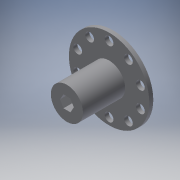
# Autodesk Inventor part: clutch plate
Saved by Autodesk Inventor 2017 (Build 210142000, 142)
## iProperties
Created: 2017-11-23
Part Number: clutch plate
Material: Generic
Document SubType Name: Modeling
Designer: prakh
Density: 1 g/cm^3
Appearance: Default
Author: prakh
Autodesk Inventor part; units mm, degrees
ref_plane "YZ Plane" through (0, 0, 0) normal (1, 0, 0) x (0, 1, 0)
ref_plane "XZ Plane" through (0, 0, 0) normal (0, 1, 0) x (-1, 0, 0)
ref_plane "XY Plane" through (0, 0, 0) normal (0, 0, 1) x (1, 0, 0)
sketch "Sketch1" plane through (0, 0, 0) normal (0, 0, 1) x (1, 0, 0)
  circle A0 centre (0, 0) radius 31.75
  circle A1 centre (0, 26.0608) radius 3.429
  line L0 (2.7496, 4.7625) -> (5.4993, 0)
  line L1 (5.4993, 0) -> (2.7496, -4.7625)
  line L2 (2.7496, -4.7625) -> (-2.7496, -4.7625)
  line L3 (-2.7496, -4.7625) -> (-5.4993, 0)
  line L4 (-5.4993, 0) -> (-2.7496, 4.7625)
  line L5 (-2.7496, 4.7625) -> (2.7496, 4.7625)
  circle A2 centre (-15.3182, 21.0836) radius 3.429
  circle A3 centre (-24.7853, 8.0532) radius 3.429
  circle A4 centre (-24.7853, -8.0532) radius 3.429
  circle A5 centre (-15.3182, -21.0836) radius 3.429
  circle A6 centre (0, -26.0608) radius 3.429
  circle A7 centre (15.3182, -21.0836) radius 3.429
  circle A8 centre (24.7853, -8.0532) radius 3.429
  circle A9 centre (24.7853, 8.0532) radius 3.429
  circle A10 centre (15.3182, 21.0836) radius 3.429
  dimension "d0" = 6.858
  dimension "d1" = 9.525
  dimension "d4" = 360
  dimension "d8" = 63.5
  constraints: 12 end point, 11 centre point, 2 coincident, 34 other
  measures "d0" diameter of A1
  measures "d1" distance between parallel lines of L5 L2
  measures "d8" diameter of A0
extrude "Extrusion1" add sketch "Sketch1" along normal blind 3.175
sketch "Sketch2" plane through (0, 0, 3.175) normal (0, 0, 1) x (1, 0, 0)
  line L0 (5.4993, 0) -> (2.7496, -4.7625) projected
  line L1 (2.7496, -4.7625) -> (-2.7496, -4.7625) projected
  line L2 (-2.7496, -4.7625) -> (-5.4993, 0) projected
  line L3 (-5.4993, 0) -> (-2.7496, 4.7625) projected
  line L4 (-2.7496, 4.7625) -> (2.7496, 4.7625) projected
  line L5 (2.7496, 4.7625) -> (5.4993, 0) projected
  circle A0 centre (15.3182, 21.0836) radius 3.429 projected
  circle A1 centre (24.7853, 8.0532) radius 3.429 projected
  circle A2 centre (24.7853, -8.0532) radius 3.429 projected
  circle A3 centre (15.3182, -21.0836) radius 3.429 projected
  circle A4 centre (0, -26.0608) radius 3.429 projected
  circle A5 centre (-15.3182, -21.0836) radius 3.429 projected
  circle A6 centre (-24.7853, -8.0532) radius 3.429 projected
  circle A7 centre (-24.7853, 8.0532) radius 3.429 projected
  circle A8 centre (-15.3182, 21.0836) radius 3.429 projected
  circle A9 centre (0, 26.0608) radius 3.429 projected
  circle A10 centre (0, 0) radius 31.75 projected
  circle A11 centre (0, 0) radius 12.7
  dimension "d9" = 25.4
  constraints: 1 centre point, 1 coincident
  measures "d9" diameter of A11
extrude "Extrusion2" add sketch "Sketch2" along normal blind 33.3375 contours A11
body "Solid1"
